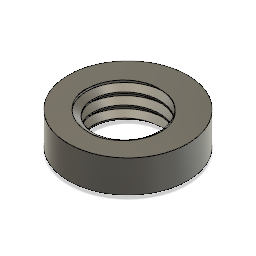
laserNut (Autodesk Fusion 360 design; units mm, degrees)
Autodesk Fusion 360 part; units mm, degrees
sketch "Sketch1" plane through (0, 0, 0) normal (0, 1, 0) x (1, 0, 0)
  circle A0 centre (0, 0) radius 9.2075
  dimension "d1" = 18.415
  measures "d1" diameter of A0
extrude "Extrude1" add sketch "Sketch1" along normal blind 5
hole "Hole1" at (0, 5, 0) direction (0, -1, 0) diameter 10.274 depth 9 tip angle 118
thread "Thread1" "ISO Metric profile 12.0 M12x1.75 6H" major diameter 12.2265 minor diameter 10.2735 pitch 1.75 angle 60 modelled right hand crest width 0.2188 on face at (0.2561, 3.3333, 5.1306) crest through (0, 5.9844, 5.1368)
